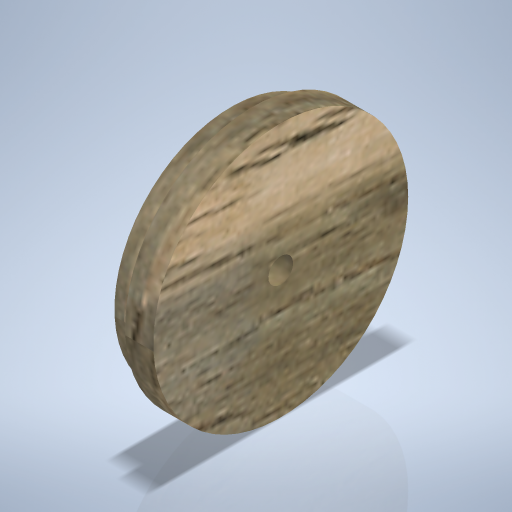
# Autodesk Inventor part: lid
Saved by Autodesk Inventor 2024 (Build 280153000, 153)
## iProperties
Created: 2024-04-24
Part Number: lid
Material: Kupfer, Guss
Document SubType Name: Modeling
Designer: ffogue
Density: 8.94 g/cm^3
Appearance: Treibholz
Author: ffogue
Autodesk Inventor part; units mm, degrees
ref_plane "YZ Plane" through (0, 0, 0) normal (1, 0, 0) x (0, 1, 0)
ref_plane "XZ Plane" through (0, 0, 0) normal (0, 1, 0) x (-1, 0, 0)
ref_plane "XY Plane" through (0, 0, 0) normal (0, 0, 1) x (1, 0, 0)
sketch "Skizze1" plane through (0, 0, 0) normal (0, 0, 1) x (1, 0, 0)
  line L0 (0, 0) -> (33.3235, 0)
  line L1 (0, 0) -> (0, 16.5)
  line L2 (0, 16.5) -> (3, 16.5)
  line L3 (3, 16.5) -> (3, 18)
  line L4 (3, 18) -> (7, 18)
  line L5 (7, 18) -> (7, 0)
  dimension "d0" = 3
  dimension "d1" = 4
  dimension "d2" = 36
  dimension "d3" = 33
  constraints: 12 end point, 4 perpendicular, 1 horizontal, 1 point on line, 1 vertical
  measures "d0" distance between parallel lines of L3 L1
  measures "d1" distance between parallel lines of L5 L3
  measures "d2" diameter of L4 L0
  measures "d3" diameter of L2 L0
revolve "Umdrehung1" add sketch "Skizze1" angle 360 about axis through (0, 0, 0) along (1, 0, 0)
sketch "Skizze2" plane through (7, 0, 0) normal (1, 0, 0) x (0, 0, -1)
  circle A0 centre (0, 0) radius 1.75
  dimension "d5" = 3.5
  constraints: 1 centre point, 1 coincident
  measures "d5" diameter of A0
extrude "Extrusion1" cut sketch "Skizze2" against normal up to surface (7 mm away)
